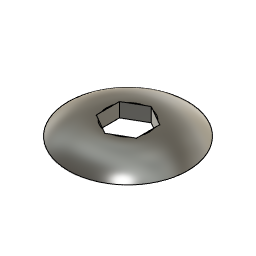
Bolt-Cap_F3-01_008 (Autodesk Fusion 360 design; units mm, degrees)
Autodesk Fusion 360 part; units mm, degrees
sketch "Sketch1" plane through (0, 0, 0) normal (0, 0, 1) x (1, 0, 0)
  line L0 (0, 6) -> (-5.1962, 3)
  line L1 (-5.1962, 3) -> (-5.1962, -3)
  line L2 (-5.1962, -3) -> (0, -6)
  line L3 (0, -6) -> (5.1962, -3)
  line L4 (5.1962, -3) -> (5.1962, 3)
  line L5 (5.1962, 3) -> (0, 6)
  dimension "d1" = 6
  measures "d1" distance of L0.start origin
extrude "Extrude1" add sketch "Sketch1" along normal blind 10 makes body 1
cylinder "CylinderPrimitive1" add diameter 38 height 4.5 placed x (1, 0, 0) y (0, 1, 0) z (0, 0, 1) at (0, 0, 0) separate body makes body 2
scale "Scale1" factor 1.23 about (0, 0, 0) bodies 1
fillet "Fillet1" radius 19 1 edges at (-17.7142, -6.8707, 4.5) on bodies 2
combine "Combine1" operation cut target body 2 tool bodies 1
